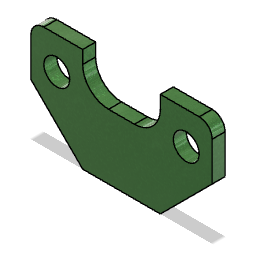
3d05 v1 (Autodesk Fusion 360 design; units mm, degrees)
Autodesk Fusion 360 part; units mm, degrees
sketch "Sketch1" plane through (0, 0, 0) normal (0, 0, 1) x (1, 0, 0)
  line L0 (20, 0) -> (50, 0)
  line L1 (70, 20) -> (70, 35)
  line L2 (0, 35) -> (0, 20)
  line L3 (70, 20) -> (50, 0)
  line L4 (20, 0) -> (0, 20)
  arc A0 (5, 40) -> (0, 35) centre (5, 35) ccw
  arc A1 (70, 35) -> (65, 40) centre (65, 35) ccw
  circle A2 centre (10, 27.5) radius 5
  circle A3 centre (60, 27.5) radius 5
  line L5 (-87.2465, 27.5) -> (87.2465, 27.5) construction
  line L6 (60, 39.9875) -> (60, -19.9875) construction
  line L7 (10, 40.8142) -> (10, -20.8142) construction
  line L8 (20, 40) -> (20, 35)
  line L9 (30, 25) -> (40, 25)
  line L10 (50, 40) -> (50, 35)
  arc A4 (40, 25) -> (50, 35) centre (40, 35) ccw
  arc A5 (35, 26.3397) -> (36.6144, 27.5) centre (30, 35) ccw
  arc A6 (33.3856, 27.5) -> (35, 26.3397) centre (40, 35) ccw
  arc A7 (20, 35) -> (30, 25) centre (30, 35) ccw
  line L11 (65, 40) -> (50, 40)
  line L12 (20, 40) -> (5, 40)
  point P0 (70, 0)
  point P1 (0, 40)
  dimension "d1" = 70
  dimension "d2" = 20
  dimension "d3" = 20
  dimension "d4" = 20
  dimension "d5" = 20
  dimension "d6" = 40
  dimension "d7" = 5
  dimension "d8" = 5
  dimension "d9" = 10
  dimension "d10" = 10
  dimension "d12" = 10
  dimension "d13" = 10
  dimension "d14" = 20
  dimension "d16" = 20
  dimension "d17" = 20
  dimension "d20" = 25
  dimension "d22" = 10
  dimension "d25" = 5
  dimension "d26" = 10
  dimension "d27" = 10
  constraint horizontal L0
  constraint perpendicular L0 L1
  constraint perpendicular L1 L11
  constraint perpendicular L0 L2
  constraint coincident P0 L1
  constraint coincident P0 L0
  constraint coincident origin L0
  constraint coincident origin L2
  constraint coincident P1 L11
  constraint coincident P1 L2
  constraint tangent A0 L11
  constraint tangent L2 A0
  constraint tangent L1 A1
  constraint tangent A1 L11
  constraint horizontal L5
  constraint midpoint L2 L5
  constraint vertical L6
  constraint parallel L6 L7
  constraint midpoint L4 L7
  constraint midpoint L3 L6
  constraint coincident A2.centre L5
  constraint coincident A3.centre L5
  constraint perpendicular L5 L10
  constraint vertical L8
  constraint tangent L8 A5
  constraint coincident L8.start L11
  constraint coincident L8.end A5
  constraint coincident L5 A5.end
  constraint coincident L5 A6.start
  constraint collinear L11 L12
  measures "d1" distance of origin P0
  measures "d2" distance of P0 L1.start
  measures "d3" distance of P0 L0.end
  measures "d4" distance of origin L0.start
  measures "d5" distance of origin L2.end
  measures "d6" distance of origin P1
  measures "d7" radius of A0
  measures "d8" radius of A1
  measures "d9" diameter of A2
  measures "d10" diameter of A3
  measures "d12" horizontal distance of L0.end A3.centre
  measures "d13" horizontal distance of L0.start A2.centre
  measures "d14" diameter of A5
  measures "d16" distance of L1 L10
  measures "d17" distance of L2 L8
  measures "d20" distance of L0 L9
  measures "d22" distance of A4.centre A5.centre
  measures "d25" vertical distance of L8.start A5.centre
  measures "d26" distance of L9 A5.centre
  measures "d27" distance of A4.centre A5.centre
extrude "Extrude1" add sketch "Sketch1" along normal blind 5
